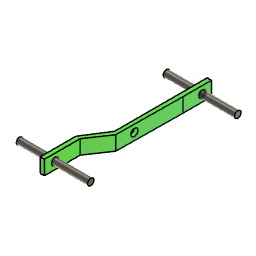
suspencion armada v1 (Autodesk Fusion 360 archive; units mm, degrees)
design "brazo de suspencion"
Autodesk Fusion 360 part; units mm, degrees
sketch "Sketch1" plane through (0, 0, 0) normal (0, 0, 1) x (1, 0, 0)
  line L0 (0, 0) -> (3, 0)
  line L1 (3, 0) -> (3, 25)
  line L2 (3, 25) -> (-15, 25) construction
  line L3 (-6.9872, 39.9752) -> (-9.4831, 38.3106)
  line L4 (3, 25) -> (13.0655, 39.9227)
  line L5 (3, 25) -> (21, 25) construction
  line L6 (13.0655, 39.9227) -> (10.5784, 41.6003)
  line L7 (10.5784, 41.6003) -> (0, 25)
  line L8 (10.5784, 41.6003) -> (10.5784, 86.6003)
  line L9 (10.5784, 86.6003) -> (13.5784, 86.6003)
  line L10 (13.5784, 86.6003) -> (13.0655, 39.9227)
  line L11 (0, 25) -> (0, 0)
  dimension "d1" = 3
  dimension "d2" = 25
  dimension "d6" = 56
  dimension "d7" = 18
  dimension "d8" = 3
  dimension "d9" = 45
  dimension "d10" = 3
  constraint coincident L0.start L11.end
  constraint horizontal L0
  constraint perpendicular L0 L1
  constraint horizontal L2
  constraint horizontal L5
  constraint perpendicular L4 L6
  constraint coincident L2 L7.end
  constraint vertical L8
  constraint perpendicular L8 L9
  constraint perpendicular L0 L11
  measures "d1" distance of L0.start L0.end
  measures "d2" distance of L0.end L1.end
  measures "d6" angle of L4 L5
  measures "d7" distance of L1.end L4.end
  measures "d8" distance of L4.end L6.end
  measures "d9" distance of L6.end L8.end
  measures "d10" distance of L8.end L9.end
extrude "Extrude1" add sketch "Sketch1" along normal blind 10 makes body 1
sketch "Sketch2" plane through (3, 0, 0) normal (1, 0, 0) x (0, 1, 0)
  line L0 (0, 0) -> (25, 0)
  line L1 (25, 0) -> (25, 10)
  line L2 (25, 10) -> (0, 10)
  line L3 (0, 10) -> (0, 0)
  line L4 (0, 5) -> (7.5, 5)
  circle A0 centre (7.5, 5) radius 2.5
  dimension "d13" = 7.5
  dimension "d14" = 5
  constraint midpoint L3 L4.start
  constraint perpendicular L3 L4
  constraint coincident L4.end A0.centre
  measures "d13" distance of L4.start L4.end
  measures "d14" diameter of A0
extrude "Extrude2" cut sketch "Sketch2" against normal blind 17 contours A0 bodies 1
sketch "Sketch3" plane through (12.6253, -0.1387, 0) normal (0.99994, -0.010987, 0) x (0.010987, 0.99994, 0)
  line L0 (40.0638, 0) -> (86.7442, 0)
  line L1 (86.7442, 0) -> (86.7442, 10)
  line L2 (86.7442, 10) -> (40.0638, 10)
  line L3 (40.0638, 10) -> (40.0638, 0)
sketch "Sketch4" plane through (0, 0, 0) normal (1, 0, 0) x (0, 1, 0)
sketch "Sketch5" plane through (12.6253, -0.1387, 0) normal (0.99994, -0.010987, 0) x (0.010987, 0.99994, 0)
  circle A0 centre (53, 5) radius 2.5
  dimension "d19" = 5
  measures "d19" diameter of A0
extrude "Extrude3" cut sketch "Sketch5" against normal blind 10 bodies 1
sketch "Sketch6" plane through (0, 0, 0) normal (0, 0, -1) x (1, 0, 0)
  line L0 (0, -25) -> (10.5784, -41.6003)
  line L1 (10.5784, -41.6003) -> (10.5784, -86.6003)
  line L2 (10.5784, -86.6003) -> (13.5784, -86.6003)
  line L3 (13.5784, -86.6003) -> (13.0655, -39.9227)
  line L4 (13.0655, -39.9227) -> (3, -25)
  line L5 (3, -25) -> (3, 0)
  line L6 (3, 0) -> (0, 0)
  line L7 (0, 0) -> (0, -25)
  line L8 (13.5784, -86.6003) -> (13.5784, -106.6003)
  line L9 (13.5784, -106.6003) -> (10.5784, -106.6003)
  line L10 (10.5784, -106.6003) -> (10.5784, -86.6003)
  dimension "d22" = 20
  dimension "d23" = 3
  constraint coincident L2.end L3.start
  constraint perpendicular L2 L8
  constraint perpendicular L8 L9
  constraint coincident L1.end L2.start
  measures "d22" distance of L2.end L8.end
  measures "d23" distance of L8.end L9.end
extrude "Extrude4" add sketch "Sketch6" against normal blind 10 contours L2 L8 L9 L10 bodies 1
sketch "Sketch7" plane through (13.5784, 0, 0) normal (1, 0, 0) x (0, 1, 0)
  line L0 (86.6003, 0) -> (106.6003, 0)
  line L1 (106.6003, 0) -> (106.6003, 10)
  line L2 (106.6003, 10) -> (86.6003, 10)
  line L3 (86.6003, 10) -> (86.6003, 0)
  circle A0 centre (100, 5) radius 2.5
  dimension "d26" = 5
  measures "d26" diameter of A0
extrude "Extrude5" cut sketch "Sketch7" against normal blind 10 contours A0 bodies 1
sketch "Sketch8" plane through (13.5784, 0, 0) normal (1, 0, 0) x (0, 1, 0)
  circle A0 centre (100, 5) radius 2.5
  line L0 (86.6003, 0) -> (106.6003, 0)
  line L1 (106.6003, 0) -> (106.6003, 10)
  line L2 (106.6003, 10) -> (86.6003, 10)
  line L3 (86.6003, 10) -> (86.6003, 0)
  circle A1 centre (100, 5) radius 2.3
  dimension "d31" = 4.6
  constraint concentric A0 A1
  measures "d31" diameter of A1
extrude "Extrude6" add sketch "Sketch8" against normal blind 30 contours A0 | A1 bodies 1
extrude "Extrude7" add sketch "Sketch8" along normal blind 25 and the other way blind 25 separate body contours A1 makes body 2
sketch "Sketch9" plane through (3, 0, 0) normal (1, 0, 0) x (0, 1, 0)
  circle A0 centre (7.5, 5) radius 2.5
  line L0 (0, 0) -> (25, 0)
  line L1 (25, 0) -> (25, 10)
  line L2 (25, 10) -> (0, 10)
  line L3 (0, 10) -> (0, 0)
  circle A1 centre (7.5, 5) radius 2.25
  dimension "d36" = 4.5
  constraint concentric A0 A1
  measures "d36" diameter of A1
extrude "Extrude8" add sketch "Sketch9" along normal blind -25 and the other way blind -25 separate body contours A1 makes body 3
delete_face "DeleteFace1" 1 faces at (-7.4216, 102.4876, 4.7511) on bodies 1
